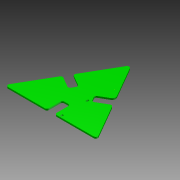
# Autodesk Inventor part: base
Saved by Autodesk Inventor 2012 (Build 160160000, 160)
## iProperties
Created: 2013-10-01
Part Number: base
Material: Default
Document SubType Name: Modeling
Designer: Nick
Density: 1 g/cm^3
Author: Nick
Autodesk Inventor part; units mm, degrees
ref_plane "YZ Plane" through (0, 0, 0) normal (1, 0, 0) x (0, 1, 0)
ref_plane "XZ Plane" through (0, 0, 0) normal (0, 1, 0) x (-1, 0, 0)
ref_plane "XY Plane" through (0, 0, 0) normal (0, 0, 1) x (1, 0, 0)
sketch "Sketch1" plane through (0, 0, 0) normal (0, 0, 1) x (1, 0, 0)
  line L0 (66.2158, -98.8819) -> (-113.7842, -98.8819) construction
  line L1 (-113.7842, -98.8819) -> (-23.7842, 57.0027) construction
  line L2 (-23.7842, 57.0027) -> (-23.7842, -98.8819) construction
  line L3 (66.2158, -98.8819) -> (-68.7842, -20.9396) construction
  line L4 (-31.2842, -98.8819) -> (-31.2842, -68.8819)
  line L5 (-31.2842, -68.8819) -> (-16.2842, -68.8819)
  line L6 (-16.2842, -68.8819) -> (-16.2842, -98.8819)
  line L7 (-65.0342, -14.4444) -> (-39.0535, -29.4444)
  line L8 (-39.0535, -29.4444) -> (-46.5535, -42.4348)
  line L9 (-46.5535, -42.4348) -> (-72.5342, -27.4348)
  line L10 (-72.5342, -27.4348) -> (-113.7842, -98.8819)
  line L11 (-31.2842, -98.8819) -> (-113.7842, -98.8819)
  line L12 (-16.2842, -98.8819) -> (66.2158, -98.8819)
  line L13 (-23.7842, 57.0027) -> (-65.0342, -14.4444)
  line L14 (-113.7842, -98.8819) -> (21.2158, -20.9396) construction
  line L15 (-23.7842, 57.0027) -> (66.2158, -98.8819) construction
  line L16 (17.4658, -14.4444) -> (-8.515, -29.4444)
  line L17 (-8.515, -29.4444) -> (-1.015, -42.4348)
  line L18 (-1.015, -42.4348) -> (24.9658, -27.4348)
  line L19 (-23.7842, 57.0027) -> (17.4658, -14.4444)
  line L20 (24.9658, -27.4348) -> (66.2158, -98.8819)
  point P0 (-23.7842, -46.9203)
  point P1 (-23.7842, -46.9203)
  dimension "d3" = 180
  dimension "d6" = 7.5
  dimension "d7" = 15
  dimension "d8" = 30
  dimension "d9" = 15
  dimension "d10" = 7.5
  dimension "d16" = 30
  dimension "d18" = 15
  dimension "d19" = 7.5
  dimension "d20" = 30
  constraints: 42 end point, 11 perpendicular, 6 point on line, 3 collinear, 2 midpoint, 2 parallel, 1 coincident, 1 horizontal, 5 other
  measures "d3" distance of L1.end L0.start
  measures "d6" distance between parallel lines of L7 L3
  measures "d7" distance between parallel lines of L7 L9
  measures "d8" distance of L7.start L7.end
  measures "d9" distance of L4.end L5.end
  measures "d10" distance between parallel lines of L4 L2
  measures "d16" distance of L5.end L6.end
  measures "d18" distance of L16.end L17.end
  measures "d19" distance between parallel lines of L16 L14
  measures "d20" distance of L17.end L18.end
extrude "Extrusion2" add sketch "Sketch1" along normal blind 3
fillet "Fillet1" radius 6.75 1 edges at (17.4658, -14.4444, 1.5)
fillet "Fillet2" radius 4 14 edges at (-8.515, -29.4444, 1.5) (24.9658, -27.4348, 1.5) (-1.015, -42.4348, 1.5) (-31.2842, -98.8819, 1.5) (-31.2842, -68.8819, 1.5) (-16.2842, -98.8819, 1.5) (66.2158, -98.8819, 1.5) (-16.2842, -68.8819, 1.5) (-113.7842, -98.8819, 1.5) (-65.0342, -14.4444, 1.5) (-39.0535, -29.4444, 1.5) (-46.5535, -42.4348, 1.5) (-72.5342, -27.4348, 1.5) (-23.7842, 57.0027, 1.5)
sketch "Sketch3" plane through (0, 0, 3) normal (0, 0, 1) x (1, 0, 0)
  line L0 (59.2876, -98.8819) -> (-12.2842, -98.8819) projected
  line L1 (-8.2842, -91.8819) -> (-5.2842, -91.8819)
  line L2 (-5.2842, -91.8819) -> (-5.2842, -96.8819)
  line L3 (-5.2842, -96.8819) -> (-8.2842, -96.8819)
  line L4 (-8.2842, -96.8819) -> (-8.2842, -91.8819)
  line L5 (-16.2842, -94.8819) -> (-16.2842, -72.8819) projected
  line L6 (-8.2842, -42.3819) -> (-5.2842, -42.3819)
  line L7 (-5.2842, -42.3819) -> (-5.2842, -47.3819)
  line L8 (-5.2842, -47.3819) -> (-8.2842, -47.3819)
  line L9 (-8.2842, -47.3819) -> (-8.2842, -42.3819)
  point P0 (0, 0)
  dimension "d35" = 3
  dimension "d36" = 5
  dimension "d38" = 2
  dimension "d41" = 8
  dimension "d42" = 3
  dimension "d43" = 5
  dimension "d44" = 44.5
  constraints: 16 end point, 4 parallel, 2 horizontal, 2 perpendicular, 1 vertical alignment
  measures "d35" distance of L2.end L3.end
  measures "d36" distance of L1.end L2.end
  measures "d38" distance between parallel lines of L3 L0
  measures "d41" distance between parallel lines of L5 L4
  measures "d42" distance of L7.end L8.end
  measures "d43" distance of L6.end L7.end
  measures "d44" distance between parallel lines of L8 L1
extrude "Extrusion4" cut sketch "Sketch3" against normal blind 3
equation "\"d6\" = 0.5 * d7"
equation "\"d9\" = d7"
equation "\"d10\" = d6"
equation "\"d16\" = d15"
equation "\"d18\" = d7"
equation "\"d19\" = d6"
equation "\"d20\" = d16"
equation "\"d15\" = d8"
body "Solid2"
